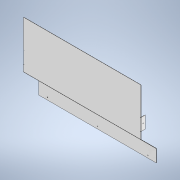
# Autodesk Inventor part: Tapa_blanca_trasera
Saved by Autodesk Inventor 2021 (Build 250183000, 183)
## iProperties
Created: 2021-04-16
Part Number: Tapa_blanca_trasera
Material: Acero AISI 1006 85 LC
Document SubType Name: Chapa
Designer: Admin
Density: 7.872 g/cm^3
Sheet Metal Rule: Por defecto_mm
Appearance: Blanco
Mass: 1172.3 g
Surface Area: 3933.58 cm^2
Volume: 148.92 cm^3
Flat Pattern Width: 36.7334 cm
Flat Pattern Length: 56.4382 cm
Flat Pattern Area: 2073.17 cm^2
Sheet Metal Width: 367,334 mm
Sheet Metal Length: 564,382 mm
Sheet Metal Area: 207316,723 mm^2
Author: Admin
Autodesk Inventor part; units mm, degrees
ref_plane "YZ Plane" through (0, 0, 0) normal (1, 0, 0) x (0, 1, 0)
ref_plane "XZ Plane" through (0, 0, 0) normal (0, 1, 0) x (-1, 0, 0)
ref_plane "XY Plane" through (0, 0, 0) normal (0, 0, 1) x (1, 0, 0)
sketch "Boceto1" plane through (0, 0, 0) normal (0, 0, 1) x (1, 0, 0)
  line L0 (0, 0) -> (527.58, 0)
  line L1 (0, 0) -> (0, 56.2)
  line L2 (527.58, 0) -> (527.58, 56.2)
  line L3 (527.58, 56.2) -> (0, 56.2)
  dimension "d0" = 527.58
  dimension "d1" = 56.2
  dimension "d2" = 56.2
  measures "d0" distance of L0.start L0.end
  measures "d1" distance of L0.start L1.end
  measures "d2" distance of L0.end L2.end
extrude "Placa1" add sketch "Boceto1" along normal blind 0.92
sketch "Boceto2" plane through (0, 55.5486, 0.6496) normal (0, 0.7080934, -0.7061188) x (-1, 0, 0)
  line L0 (-527.58, 0) -> (0, 0)
  line L1 (0, 0) -> (0, 98.854)
  line L2 (0, 98.854) -> (-527.58, 98.854)
  line L3 (-527.58, 98.854) -> (-527.58, 0)
  constraints: 6 end point, 1 horizontal, 1 perpendicular, 1 vertical
edge flange "Pestaña1" height 98.854 angle 45.08 thickness 0.92 bend radius 0.92 thickness toward (0, 0.7080934, -0.7061188) relief straight relief width 0.92 relief depth 0.46 edges at (263.79, 56.2, 0.92) wall of the first edge with corners at (527.58, 55.5486, 0.6496) (0, 55.5486, 0.6496) (0, 125.3512, 70.6475) (527.58, 125.3512, 70.6475)
bend "Doblez1"
corner "Esquina1"
sketch "Boceto3" plane through (0, 125.3512, 69.7275) normal (0, 0, 1) x (-1, 0, 0)
  line L0 (-527.58, 0) -> (0, 0)
  line L1 (0, 0) -> (0, 213.25)
  line L2 (0, 213.25) -> (-527.58, 213.25)
  line L3 (-527.58, 213.25) -> (-527.58, 0)
  constraints: 6 end point, 1 horizontal, 1 perpendicular, 1 vertical
edge flange "Pestaña2" height 213.25 angle -45.08 thickness 0.92 bend radius 0.92 thickness toward (0, 0, 1) relief straight relief width 0.92 relief depth 0.46 edges at (263.79, 125.3512, 70.6475) wall of the first edge with corners at (527.58, 125.3512, 69.7275) (0, 125.3512, 69.7275) (0, 338.6012, 69.7275) (527.58, 338.6012, 69.7275)
bend "Doblez2"
corner "Esquina2"
sketch "Boceto4" plane through (0, 126.1149, 70.6475) normal (-1, 0, 0) x (0, 0, 1)
  line L0 (0, 0) -> (0, 212.4863)
  line L1 (0, 85.3289) -> (-20, 85.3289)
  line L2 (-20, 85.3289) -> (-20, 30.3289)
  line L3 (-20, 30.3289) -> (0, 30.3289)
  line L4 (0, 30.3289) -> (0, 85.3289)
  point P0 (-70.6475, -126.1149)
  dimension "d24" = 20
  dimension "d25" = 55
  measures "d24" distance of L3.end L2.end
  measures "d25" distance of L2.end L1.end
sheet face with bend "Cara2" sketch "Boceto4" thickness 0.92 toward (1, 0, 0) bend radius 0.92 relief straight relief width 0.92 relief depth 0.46
bend "Doblez3"
sketch "Boceto5" plane through (527.58, 126.1149, 69.7275) normal (1, 0, 0) x (0, 0, -1)
  line L0 (-0.92, 85.3289) -> (0, 85.3289)
  line L1 (19.08, 85.3289) -> (19.08, 30.3289)
  line L2 (-0.92, 85.3289) -> (19.08, 85.3289)
  line L3 (19.08, 85.3289) -> (19.08, 30.3289)
  line L4 (19.08, 30.3289) -> (-0.92, 30.3289)
  line L5 (-0.92, 30.3289) -> (-0.92, 85.3289)
  point P0 (69.7275, -126.1149)
sheet face with bend "Cara3" sketch "Boceto5" thickness 0.92 toward (-1, 0, 0) bend radius 0.92 relief straight relief width 0.92 relief depth 0.46
bend "Doblez4"
fillet "Redondeo de esquina1" radius 1.5 1 edges at (527.58, 338.6012, 70.1875)
fillet "Redondeo de esquina2" radius 1.5 1 edges at (0, 338.6012, 70.1875)
sketch "Boceto9" plane through (0, 0, 0.92) normal (0, 0, 1) x (1, 0, 0)
  circle A0 centre (263.79, 10.8421) radius 1.45
  circle A1 centre (38.1, 10.8421) radius 1.45
  circle A2 centre (489.48, 10.8421) radius 1.45
  point P0 (0, 0)
  constraints: 3 centre point, 6 other
extrude "Extrusión1" cut sketch "Boceto9" against normal through all
sketch "Boceto10" plane through (0, 126.1149, 70.6475) normal (-1, 0, 0) x (0, 0, 1)
  circle A0 centre (-10.455, 57.8289) radius 1.45
  point P0 (-70.6475, -126.1149)
  constraints: 1 centre point, 2 other
extrude "Extrusión2" cut sketch "Boceto10" against normal through all
equation "\"d3\" = Grosor"
equation "\"d4\" = Anchura_desahogo_plegado"
equation "\"d5\" = Profundidad_desahogo_plegado"
equation "\"d6\" = Remanente_mínimo"
equation "\"d7\" = Radiodetransición"
equation "\"d10\" = Radio_pliegue"
equation "\"d11\" = Tamaño_destalonado"
equation "\"d12\" = TamañoSeparación"
equation "\"d13\" = Tamaño_de_radio_de_Jacobi"
equation "\"d14\" = Anchura_desahogo_plegado"
equation "\"d15\" = Profundidad_desahogo_plegado"
equation "\"d16\" = Remanente_mínimo"
equation "\"d17\" = Radiodetransición"
equation "\"d20\" = Radio_pliegue"
equation "\"d21\" = Tamaño_destalonado"
equation "\"d22\" = TamañoSeparación"
equation "\"d23\" = Tamaño_de_radio_de_Jacobi"
equation "\"d26\" = Radio_pliegue"
equation "\"d27\" = Anchura_desahogo_plegado"
equation "\"d29\" = Remanente_mínimo"
equation "\"d28\" = Profundidad_desahogo_plegado"
equation "\"d30\" = Radiodetransición"
equation "\"d31\" = Radio_pliegue"
equation "\"d32\" = Anchura_desahogo_plegado"
equation "\"d34\" = Remanente_mínimo"
equation "\"d33\" = Profundidad_desahogo_plegado"
equation "\"d35\" = Radiodetransición"
equation "\"Radio_pliegue\" = Grosor"
equation "\"Anchura_desahogo_plegado\" = Grosor"
equation "\"Profundidad_desahogo_plegado\" = 0.5 * Grosor"
equation "\"Tamaño_destalonado\" = 4 * Grosor"
equation "\"Remanente_mínimo\" = 2 * Grosor"
equation "\"Radiodetransición\" = Radio_pliegue"
equation "\"Tamaño_de_radio_de_Jacobi\" = Radio_pliegue"
equation "\"TamañoSeparación\" = Grosor"
equation "\"Grosor\" = 0.92"
